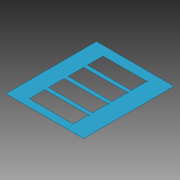
# Autodesk Inventor part: UNLHEP-14-01-P-005_ModuleStencil
Saved by Autodesk Inventor 2013 (Build 170138000, 138)
## iProperties
Created: 2014-01-06
Part Number: UNLHEP-14-01-P-005_ModuleStencil
Material: Stahl
Document SubType Name: Modeling
Designer: Frank Meier
Density: 7.85 g/cm^3
Project: UNL Pixel Phase I
Mass: 8.03712 g
Surface Area: 206.034 cm^2
Volume: 1.02384 cm^3
Author: Frank Meier
Revision Number: 00
Autodesk Inventor part; units mm, degrees
ref_plane "YZ Plane" through (0, 0, 0) normal (1, 0, 0) x (0, 1, 0)
ref_plane "XZ Plane" through (0, 0, 0) normal (0, 1, 0) x (-1, 0, 0)
ref_plane "XY Plane" through (0, 0, 0) normal (0, 0, 1) x (1, 0, 0)
ref_plane "Arbeitsebene1" through (0, 0, 0) normal (0, 0, 1) x (1, 0, 0)
sketch "Skizze2" plane through (0, 0, 0) normal (0, 0, 1) x (1, 0, 0)
  line L0 (-60, -70) -> (60, -70) projected
  line L1 (60, -70) -> (60, 70) projected
  line L2 (60, 70) -> (-60, 70) projected
  line L3 (-60, 70) -> (-60, -70) projected
  circle A0 centre (-28.35, -39.72) radius 0.75 projected
  circle A1 centre (-28.35, -50.28) radius 0.75 projected
  circle A2 centre (-20.25, -50.28) radius 0.75 projected
  circle A3 centre (-12.15, -50.28) radius 0.75 projected
  circle A4 centre (-4.05, -50.28) radius 0.75 projected
  circle A5 centre (4.05, -50.28) radius 0.75 projected
  circle A6 centre (12.15, -50.28) radius 0.75 projected
  circle A7 centre (20.25, -50.28) radius 0.75 projected
  circle A8 centre (28.35, -50.28) radius 0.75 projected
  circle A9 centre (28.35, -39.72) radius 0.75 projected
  circle A10 centre (20.25, -39.72) radius 0.75 projected
  circle A11 centre (12.15, -39.72) radius 0.75 projected
  circle A12 centre (4.05, -39.72) radius 0.75 projected
  circle A13 centre (-4.05, -39.72) radius 0.75 projected
  circle A14 centre (-12.15, -39.72) radius 0.75 projected
  circle A15 centre (-20.25, -39.72) radius 0.75 projected
  circle A16 centre (-28.35, -9.72) radius 0.75 projected
  circle A17 centre (-28.35, -20.28) radius 0.75 projected
  circle A18 centre (-20.25, -20.28) radius 0.75 projected
  circle A19 centre (-12.15, -20.28) radius 0.75 projected
  circle A20 centre (-4.05, -20.28) radius 0.75 projected
  circle A21 centre (4.05, -20.28) radius 0.75 projected
  circle A22 centre (12.15, -20.28) radius 0.75 projected
  circle A23 centre (20.25, -20.28) radius 0.75 projected
  circle A24 centre (28.35, -20.28) radius 0.75 projected
  circle A25 centre (28.35, -9.72) radius 0.75 projected
  circle A26 centre (20.25, -9.72) radius 0.75 projected
  circle A27 centre (12.15, -9.72) radius 0.75 projected
  circle A28 centre (4.05, -9.72) radius 0.75 projected
  circle A29 centre (-4.05, -9.72) radius 0.75 projected
  circle A30 centre (-12.15, -9.72) radius 0.75 projected
  circle A31 centre (-20.25, -9.72) radius 0.75 projected
  circle A32 centre (-28.35, 20.28) radius 0.75 projected
  circle A33 centre (-28.35, 9.72) radius 0.75 projected
  circle A34 centre (-20.25, 9.72) radius 0.75 projected
  circle A35 centre (-12.15, 9.72) radius 0.75 projected
  circle A36 centre (-4.05, 9.72) radius 0.75 projected
  circle A37 centre (4.05, 9.72) radius 0.75 projected
  circle A38 centre (12.15, 9.72) radius 0.75 projected
  circle A39 centre (20.25, 9.72) radius 0.75 projected
  circle A40 centre (28.35, 9.72) radius 0.75 projected
  circle A41 centre (28.35, 20.28) radius 0.75 projected
  circle A42 centre (20.25, 20.28) radius 0.75 projected
  circle A43 centre (12.15, 20.28) radius 0.75 projected
  circle A44 centre (4.05, 20.28) radius 0.75 projected
  circle A45 centre (-4.05, 20.28) radius 0.75 projected
  circle A46 centre (-12.15, 20.28) radius 0.75 projected
  circle A47 centre (-20.25, 20.28) radius 0.75 projected
  circle A48 centre (-28.35, 50.28) radius 0.75 projected
  circle A49 centre (-20.25, 50.28) radius 0.75 projected
  circle A50 centre (-12.15, 50.28) radius 0.75 projected
  circle A51 centre (-4.05, 50.28) radius 0.75 projected
  circle A52 centre (4.05, 50.28) radius 0.75 projected
  circle A53 centre (12.15, 50.28) radius 0.75 projected
  circle A54 centre (20.25, 50.28) radius 0.75 projected
  circle A55 centre (28.35, 50.28) radius 0.75 projected
  circle A56 centre (28.35, 39.72) radius 0.75 projected
  circle A57 centre (20.25, 39.72) radius 0.75 projected
  circle A58 centre (12.15, 39.72) radius 0.75 projected
  circle A59 centre (4.05, 39.72) radius 0.75 projected
  circle A60 centre (-4.05, 39.72) radius 0.75 projected
  circle A61 centre (-12.15, 39.72) radius 0.75 projected
  circle A62 centre (-20.25, 39.72) radius 0.75 projected
  circle A63 centre (-28.35, 39.72) radius 0.75 projected
  point P0 (0, 0)
extrude "Extrusion1" add sketch "Skizze2" along normal blind 0.1 contours L3 L2 L1 L0 | A0 | A1 | A2 | A3 | A4 | A5 | A6 | A7 | A8 | A9 | A10 | A11 | A12 | A13 | A14 | A15 | A16 | A17 | A18 | A19 | A20 | A21 | A22 | A23 | A24 | A25 | A26 | A27 | A28 | A29 | A30 | A31 | A32 | A33 | A34 | A35 | A36 | A37 | A38 | A39 | A40 | A41 | A42 | A43 | A44 | A45 | A46 | A47 | A48 | A49 | A50 | A51 | A52 | A53 | A54 | A55 | A56 | A57 | A58 | A59 | A60 | A61 | A62 | A63
sketch "Skizze3" plane through (0, 0, 0.1) normal (0, 0, 1) x (1, 0, 0)
  line L0 (32.4, 55.58) -> (-32.4, 55.58) projected
  line L1 (-32.4, 55.58) -> (-32.4, 34.42) projected
  line L2 (-32.4, 34.42) -> (32.4, 34.42) projected
  line L3 (32.4, 34.42) -> (32.4, 55.58) projected
  line L4 (32.4, 55.58) -> (-35.4, 55.58)
  line L5 (-35.4, 55.58) -> (-35.4, 31.42)
  line L6 (-35.4, 31.42) -> (32.4, 31.42)
  line L7 (32.4, 31.42) -> (32.4, 55.58)
  circle A0 centre (32.4, 55.58) radius 1
  point P0 (0, 0)
  dimension "d5" = 3
  dimension "d6" = 3
  dimension "d7" = 2
  constraints: 8 end point, 2 parallel, 1 centre point, 1 coincident, 1 horizontal, 1 perpendicular
  measures "d5" distance between parallel lines of L5 L1
  measures "d6" distance between parallel lines of L2 L6
  measures "d7" diameter of A0
extrude "Extrusion2" cut sketch "Skizze3" against normal through all
pattern_linear "Rechteckige Anordnung1" count 4 spacing 30 along (0, -1, 0) of "Extrusion2"
